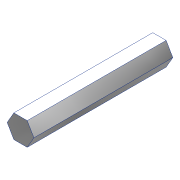
# Autodesk Inventor part: Axle
Saved by Autodesk Inventor 2020 (Build 240168000, 168)
## iProperties
Created: 2019-12-31
Part Number: Axle
Material: Aluminum 6061
Document SubType Name: Modeling
Designer: pchild
Density: 2.7 g/cm^3
Appearance: Aluminum - Flat
Author: pchild
Autodesk Inventor part; units mm, degrees
ref_plane "YZ Plane" through (0, 0, 0) normal (1, 0, 0) x (0, 1, 0)
sketch "Sketch3" plane through (0, 0, 0) normal (0, 0, 1) x (1, 0, 0)
  circle A0 centre (0, 0) radius 6.35
  dimension "d6" = 12.7
  constraints: 1 centre point, 1 coincident
  measures "d6" diameter of A0
extrude "roundShaft" [suppressed]
sketch "Sketch4" plane through (0, 0, 0) normal (0, 0, 1) x (1, 0, 0)
  line L0 (-3.6662, -6.35) -> (-7.3323, 0)
  line L1 (-7.3323, 0) -> (-3.6662, 6.35)
  line L2 (-3.6662, 6.35) -> (3.6662, 6.35)
  line L3 (3.6662, 6.35) -> (7.3323, 0)
  line L4 (7.3323, 0) -> (3.6662, -6.35)
  line L5 (3.6662, -6.35) -> (-3.6662, -6.35)
  point P0 (0, 0)
  point P1 (0, 0)
  dimension "d9" = 12.7
  constraints: 12 end point, 1 coincident, 1 horizontal, 13 other
  measures "d9" distance between parallel lines of L2 L5
extrude "hexShaft" add sketch "Sketch4" along normal blind 76.2
sketch "Sketch5" plane through (0, 0, 0) normal (1, 0, 0) x (0, 1, 0)
  line L0 (0, 0) -> (6.1468, 0)
  line L1 (6.1468, 0) -> (6.1468, -1.016)
  line L2 (6.1468, -1.016) -> (0, -1.016)
  line L3 (0, -1.016) -> (0, 0)
  line L4 (0, -1.016) -> (6.35, -1.016)
  line L5 (6.35, -1.016) -> (6.35, 0)
  line L6 (6.35, 0) -> (0, 0)
  line L7 (0, 0) -> (0, -1.016)
  line L8 (0, -1.2192) -> (0, 0.2032) projected
  point P0 (6.1468, -1.016)
  dimension "d12" = 6.1468
  dimension "d13" = 6.35
  dimension "d14" = 0
  dimension "d15" = 1.016
  constraints: 16 end point, 4 parallel, 2 horizontal, 2 perpendicular
  measures "d12" distance between parallel lines of L1 L3
  measures "d13" distance between parallel lines of L5 L7
  measures "d14" distance between parallel lines of L0 L6
  measures "d15" distance between parallel lines of L0 L2
revolve "endOneGroove" [suppressed]
ref_plane "endOnePlane" through (0, 0, 0) normal (0, 0, 1) x (1, 0, 0)
sketch "Sketch8" plane through (0, 0, 0) normal (0, 0, 1) x (1, 0, 0)
  point P0 (0, 0)
  point P1 (0, 0)
  constraints: 1 coincident
hole "endOneTap" [suppressed]
sketch "Sketch10" plane through (0, 0, 0) normal (0, 0, 1) x (1, 0, 0)
  circle A0 centre (0, 0) radius 6.35
  circle A1 centre (0, 0) radius 19.05
  dimension "d43" = 12.7
  dimension "d44" = 38.1
  constraints: 2 centre point, 2 coincident
  measures "d43" diameter of A0
  measures "d44" diameter of A1
extrude "endOneTurnDown" [suppressed]
sketch "Sketch11" plane through (0, 0, 0) normal (0, 0, 1) x (1, 0, 0)
  point P0 (0, 0)
hole "endOneMagnet" [suppressed]
ref_plane "endTwoPlane" through (0, 0, 76.2) normal (0, 0, 1) x (1, 0, 0)
sketch "Sketch6" plane through (0, 0, 0) normal (1, 0, 0) x (0, 1, 0)
  line L0 (0, 76.2) -> (6.1468, 76.2)
  line L1 (6.1468, 76.2) -> (6.1468, 77.216)
  line L2 (6.1468, 77.216) -> (0, 77.216)
  line L3 (0, 77.216) -> (0, 76.2)
  line L4 (0, 77.216) -> (6.35, 77.216)
  line L5 (6.35, 77.216) -> (6.35, 76.2)
  line L6 (6.35, 76.2) -> (0, 76.2)
  line L7 (0, 76.2) -> (0, 77.216)
  line L8 (0, -15.4432) -> (0, 92.6592) projected
  point P0 (0, 0)
  point P1 (6.1468, 77.216)
  dimension "d17" = 76.2
  dimension "d18" = 6.1468
  dimension "d19" = 6.35
  dimension "d21" = 1.016
  dimension "d61" = 76.2
  constraints: 16 end point, 4 parallel, 2 horizontal, 2 perpendicular, 1 point on line
  measures "d17" distance from line of point (0, 0) L0
  measures "d18" distance between parallel lines of L1 L3
  measures "d19" distance between parallel lines of L5 L7
  measures "d21" distance between parallel lines of L0 L2
  measures "d61" distance from line of point (0, 0) L6
revolve "endTwoGroove" [suppressed]
sketch "Sketch7" plane through (0, 0, 76.2) normal (0, 0, 1) x (1, 0, 0)
  point P0 (0, 0)
hole "endTwoTap" [suppressed]
sketch "Sketch9" plane through (0, 0, 76.2) normal (0, 0, 1) x (1, 0, 0)
  circle A0 centre (0, 0) radius 19.05
  circle A1 centre (0, 0) radius 6.35
  dimension "d39" = 38.1
  dimension "d40" = 12.7
  constraints: 2 centre point, 2 coincident
  measures "d39" diameter of A0
  measures "d40" diameter of A1
extrude "endTwoTurnDown" [suppressed]
sketch "Sketch12" plane through (0, 0, 76.2) normal (0, 0, 1) x (1, 0, 0)
  point P0 (0, 0)
hole "endTwoMagnet" [suppressed]
equation "\"d6\" = axleDiameter"
equation "\"d17\" = axleLength"
equation "\"d61\" = axleLength + e2EndLength"
equation "\"d7\" = axleLength"
equation "\"d9\" = axleDiameter"
equation "\"d10\" = axleLength"
equation "\"d12\" = -0.5 * grooveDepth + 0.5 * axleDiameter"
equation "\"d13\" = 0.5 * axleDiameter"
equation "\"d15\" = grooveWidth"
equation "\"d37\" = tapDepth"
equation "\"d43\" = axleDiameter"
equation "\"d45\" = e1EndLength + turnDownLength"
equation "\"d47\" = magnetDiameter"
equation "\"d52\" = magnetDepth"
equation "\"d18\" = -0.5 * grooveDepth + 0.5 * axleDiameter"
equation "\"d19\" = 0.5 * axleDiameter"
equation "\"d21\" = grooveWidth"
equation "\"d26\" = tapDepth"
equation "\"d30\" = tapDepth"
equation "\"d40\" = axleDiameter"
equation "\"d41\" = e2EndLength + turnDownLength"
equation "\"d54\" = magnetDiameter"
equation "\"d59\" = magnetDepth"
equation "\"axleLength\" = 76.2"
equation "\"axleDiameter\" = 12.7"
equation "\"turnDownLength\" = 7.9375"
equation "\"tapDepth\" = 6.35"
equation "\"grooveDepth\" = 0.4064"
equation "\"grooveWidth\" = 1.016"
equation "\"d24\" = axleLength + e2EndLength"
equation "\"e1EndLength\" = 0"
equation "\"e2EndLength\" = 0"
equation "\"magnetDepth\" = 9.525"
equation "\"magnetDiameter\" = 6.35"
body "Solid2"
